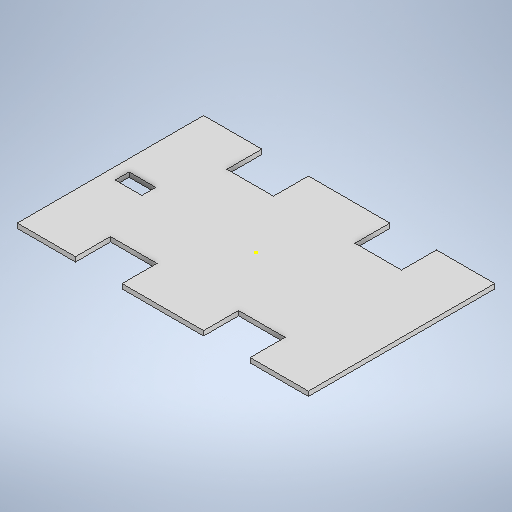
# Autodesk Inventor part: Acrylic bottom
Saved by Autodesk Inventor 2025.2 (Build 292293000, 293)
## iProperties
Created: 2025-03-13
Part Number: Acrylic bottom
Material: Generic
Document SubType Name: Modeling
Designer: CZ
Density: 1 g/cm^3
Appearance: Default
Author: CZ
Autodesk Inventor part; units mm, degrees
ref_plane "YZ Plane" through (0, 0, 0) normal (1, 0, 0) x (0, 1, 0)
ref_plane "XZ Plane" through (0, 0, 0) normal (0, 1, 0) x (-1, 0, 0)
ref_plane "XY Plane" through (0, 0, 0) normal (0, 0, 1) x (1, 0, 0)
sketch "Sketch1" plane through (0, 0, 0) normal (0, 1, 0) x (-1, 0, 0)
  point P0 (0, 0)
sketch "Sketch2" plane through (0, 0, 0) normal (0, 1, 0) x (-1, 0, 0)
  line L0 (125, 80) -> (-125, 80)
  line L1 (-125, 80) -> (-125, -80)
  line L2 (-125, -80) -> (125, -80)
  line L3 (125, -80) -> (125, 80)
  point P0 (0, 0)
  dimension "d0" = 250
  dimension "d1" = 160
  dimension "d2" = 80
  dimension "d3" = 125
  constraints: 8 end point, 2 parallel, 1 horizontal, 1 perpendicular
  measures "d0" distance between parallel lines of L1 L3
  measures "d1" distance between parallel lines of L0 L2
  measures "d2" distance from line of point (0, 0) L2
  measures "d3" distance from line of point (0, 0) L3
extrude "Extrusion1" add sketch "Sketch2" along normal blind 4
sketch "Sketch3" plane through (0, 4, 0) normal (0, 1, 0) x (1, 0, 0)
  line L0 (-75, 80) -> (-35, 80)
  line L1 (-35, 80) -> (-35, 50)
  line L2 (-35, 50) -> (-75, 50)
  line L3 (-75, 50) -> (-75, 80)
  line L4 (125, 80) -> (-125, 80) projected
  line L5 (35, 80) -> (75, 80)
  line L6 (75, 80) -> (75, 50)
  line L7 (75, 50) -> (35, 50)
  line L8 (35, 50) -> (35, 80)
  line L9 (319.9785, -5.3403) -> (359.9785, -5.3403)
  line L10 (359.9785, -5.3403) -> (359.9785, -35.3403)
  line L11 (359.9785, -35.3403) -> (319.9785, -35.3403)
  line L12 (319.9785, -35.3403) -> (319.9785, -5.3403)
  line L13 (-75, -50) -> (-35, -50)
  line L14 (-35, -50) -> (-35, -80)
  line L15 (-35, -80) -> (-75, -80)
  line L16 (-75, -80) -> (-75, -50)
  line L17 (35, -50) -> (75, -50)
  line L18 (75, -50) -> (75, -80)
  line L19 (75, -80) -> (35, -80)
  line L20 (35, -80) -> (35, -50)
  line L21 (-125, -80) -> (125, -80) projected
  line L22 (-125, 80) -> (-125, -80) projected
  line L23 (-115, 6) -> (-92, 6)
  line L24 (-92, 6) -> (-92, -6)
  line L25 (-92, -6) -> (-115, -6)
  line L26 (-115, -6) -> (-115, 6)
  point P0 (0, 0)
  point P1 (-35, 65)
  point P2 (-75, 65)
  point P3 (-55, 80)
  point P4 (75, 65)
  point P5 (160.9592, -18.931)
  point P6 (359.9785, -20.3403)
  point P7 (72.8179, -60.7416)
  point P8 (-35, -65)
  point P9 (-133.4102, -90.6871)
  point P10 (75, -65)
  point P11 (55, 80)
  point P12 (35, 65)
  point P13 (35, -65)
  point P14 (55, -80)
  point P15 (-75, -65)
  point P16 (-103.5, -6)
  point P17 (-103.5, 6)
  point P18 (-115, 0)
  point P19 (-92, 0)
  point P20 (-125, 0)
  dimension "d6" = 30
  dimension "d7" = 40
  dimension "d8" = 35
  dimension "d9" = 0
  dimension "d10" = 40
  dimension "d11" = 30
  dimension "d12" = 40
  dimension "d13" = 30
  dimension "d14" = 40
  dimension "d15" = 30
  dimension "d16" = 40
  dimension "d17" = 30
  dimension "d18" = 0
  dimension "d19" = 35
  dimension "d20" = 35
  dimension "d21" = 0
  dimension "d22" = 50
  dimension "d23" = 0
  dimension "d24" = 12
  dimension "d25" = 0
  dimension "d26" = 23
  dimension "d27" = 10
  constraints: 48 end point, 17 midpoint, 12 parallel, 6 horizontal, 6 perpendicular
  measures "d6" distance between parallel lines of L2 L0
  measures "d7" distance of point (-35, 65) point (-75, 65)
  measures "d8" horizontal distance of point (0, 0) point (-35, 65)
  measures "d9" distance from line of L4 point (-55, 80)
  measures "d10" distance from line of point (75, 65) L8
  measures "d11" distance between parallel lines of L7 L5
  measures "d12" distance from line of point (359.979, -20.34) L12
  measures "d13" distance between parallel lines of L11 L9
  measures "d14" distance from line of point (-35, -65) L16
  measures "d15" distance between parallel lines of L15 L13
  measures "d16" distance from line of point (75, -65) L20
  measures "d17" distance between parallel lines of L19 L17
  measures "d18" distance from line of L4 point (55, 80)
  measures "d19" horizontal distance of point (0, 0) point (35, 65)
  measures "d20" horizontal distance of point (0, 0) point (35, -65)
  measures "d21" distance from line of L21 point (55, -80)
  measures "d22" distance from line of L22 point (-75, -65)
  measures "d23" distance between parallel lines of L21 L15
  measures "d24" distance of point (-103.5, -6) point (-103.5, 6)
  measures "d25" vertical distance of point (0, 0) point (-115, 0)
  measures "d26" distance of point (-115, 0) point (-92, 0)
  measures "d27" distance of point (-125, 0) point (-115, 0)
extrude "Extrusion2" cut sketch "Sketch3" against normal blind 10 contours L4 L6 L7 L8 | L0 L1 L2 L3 | L20 L17 L18 L19 | L16 L13 L14 L15 | L23 L24 L25 L26
sketch "Sketch4" plane through (0, 4, 0) normal (0, 1, 0) x (1, 0, 0)
  point P0 (0, 0)
body "Solid1"
